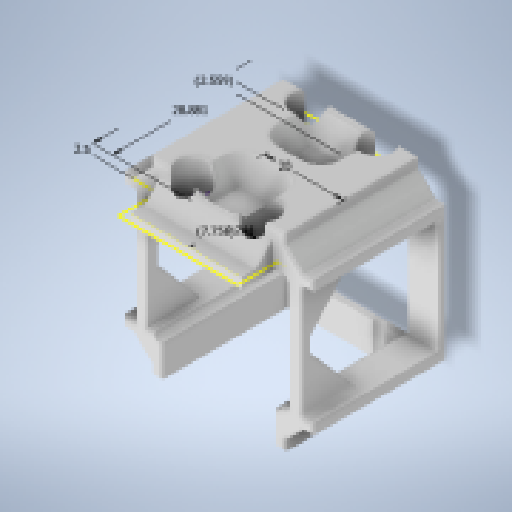
# Autodesk Inventor part: 56-spiralxy-groove-FocusToCubeAdapter
Saved by Autodesk Inventor 2024.1 (Build 281209000, 209)
## iProperties
Created: 2023-11-15
Part Number: 56-spiralxy-groove-FocusToCubeAdapter
Material: Generisch
Document SubType Name: Modeling
Designer: buchmannmartin
Density: 1 g/cm^3
Appearance: Vorgabe
Author: buchmannmartin
Autodesk Inventor part; units mm, degrees
ref_plane "YZ Plane" through (0, 0, 0) normal (1, 0, 0) x (0, 1, 0)
ref_plane "XZ Plane" through (0, 0, 0) normal (0, 1, 0) x (-1, 0, 0)
ref_plane "XY Plane" through (0, 0, 0) normal (0, 0, 1) x (1, 0, 0)
sketch "Skizze1" plane through (0, 0, 0) normal (0, 0, 1) x (1, 0, 0)
  line L0 (17.02, 23.9) -> (17.02, 21.2698) construction
  line L1 (17.02, 21.2698) -> (21.2698, 17.02) construction
  line L2 (21.2698, 17.02) -> (23.9, 17.02) construction
  line L3 (-23.9, 17.02) -> (-21.2698, 17.02) construction
  line L4 (-21.2698, 17.02) -> (-17.02, 21.2698) construction
  line L5 (-17.02, 21.2698) -> (-17.02, 23.9) construction
  line L6 (-17.02, -23.9) -> (-17.02, -21.2698) construction
  line L7 (-17.02, -21.2698) -> (-21.2698, -17.02) construction
  line L8 (-21.2698, -17.02) -> (-23.9, -17.02) construction
  line L9 (23.9, -17.02) -> (21.2698, -17.02) construction
  line L10 (21.2698, -17.02) -> (17.02, -21.2698) construction
  line L11 (17.02, -21.2698) -> (17.02, -23.9) construction
  line L12 (-14.5, 14.25) -> (14.5, 14.25)
  line L13 (16, 12.75) -> (16, -14.25)
  line L14 (14.5, -15.75) -> (-14.5, -15.75)
  line L15 (-16, -14.25) -> (-16, 12.75)
  line L16 (17.02, 23.9) -> (-17.02, 23.9) construction
  line L17 (-23.9, 17.02) -> (-23.9, -17.02) construction
  line L18 (23.9, -17.02) -> (23.9, 17.02) construction
  line L19 (17.02, -23.9) -> (-17.02, -23.9) construction
  line L20 (-16.92, 23.8) -> (-16.92, 21.2284)
  line L21 (-16.92, 21.2284) -> (-21.2284, 16.92)
  line L22 (-21.2284, 16.92) -> (-23.8, 16.92)
  line L23 (-23.8, 16.92) -> (-23.8, -16.92)
  line L24 (-23.8, -16.92) -> (-21.2284, -16.92)
  line L25 (-21.2284, -16.92) -> (-16.92, -21.2284)
  line L26 (-16.92, -21.2284) -> (-16.92, -23.8)
  line L27 (-16.92, -23.8) -> (16.92, -23.8)
  line L28 (16.92, -23.8) -> (16.92, -21.2284)
  line L29 (16.92, -21.2284) -> (21.2284, -16.92)
  line L30 (21.2284, -16.92) -> (23.8, -16.92)
  line L31 (23.8, -16.92) -> (23.8, 16.92)
  line L32 (23.8, 16.92) -> (21.2284, 16.92)
  line L33 (21.2284, 16.92) -> (16.92, 21.2284)
  line L34 (16.92, 21.2284) -> (16.92, 23.8)
  line L35 (16.92, 23.8) -> (-16.92, 23.8)
  arc A0 (16, 12.75) -> (14.5, 14.25) centre (14.5, 12.75) ccw
  arc A1 (14.5, -15.75) -> (16, -14.25) centre (14.5, -14.25) ccw
  arc A2 (-16, -14.25) -> (-14.5, -15.75) centre (-14.5, -14.25) ccw
  arc A3 (-14.5, 14.25) -> (-16, 12.75) centre (-14.5, 12.75) ccw
  point P0 (0, 0)
  point P1 (0, -15.75)
  dimension "d2" = 360
  dimension "d4" = 54.15
  dimension "d5" = 34.04
  dimension "d6" = 47.8
  dimension "d10" = 0.1
  dimension "d11" = 1.5
  dimension "d15" = 29
  dimension "d16" = 30
  dimension "d19" = 14.25
  constraints: 72 end point, 8 perpendicular, 8 point on circle, 8 tangent, 4 centre point, 4 parallel, 3 equal radius, 2 collinear, 2 horizontal, 2 vertical alignment, 1 horizontal alignment, 1 midpoint, 1 vertical, 44 other
  measures "d4" distance between parallel lines of L10 L4
  measures "d5" distance between parallel lines of L11 L6
  measures "d6" distance of L6.start L5.end
  measures "d10" distance between parallel lines of L35 L16
  measures "d11" radius of A0
  measures "d15" distance of A2.centre A1.centre
  measures "d16" distance between parallel lines of L12 L14
  measures "d19" distance from line of point (0, 0) L12
extrude "Extrusion1" add sketch "Skizze1" along normal blind 33.94
sketch "Skizze2" plane through (0, 0, 0) normal (1, 0, 0) x (0, 1, 0)
  line L0 (-15.75, 0) -> (-15.75, 33.94) construction
  line L1 (-15.75, 33.94) -> (-15.75, 38.29) construction
  line L2 (-15.75, 38.29) -> (-18.3, 38.29) construction
  line L3 (-18.3, 38.29) -> (-22.65, 33.94)
  line L4 (-22.65, 33.94) -> (-15.75, 33.94)
  line L5 (-15.75, 33.94) -> (-15.75, 41.94)
  line L6 (-15.75, 41.94) -> (-18.3, 41.94)
  line L7 (-18.3, 41.94) -> (-18.3, 38.29)
  line L8 (-0.75, 41.3732) -> (-0.75, 30.0346) construction
  line L9 (16.8, 38.29) -> (21.15, 33.94)
  line L10 (21.15, 33.94) -> (14.25, 33.94)
  line L11 (14.25, 33.94) -> (14.25, 41.94)
  line L12 (14.25, 41.94) -> (16.8, 41.94)
  line L13 (16.8, 41.94) -> (16.8, 38.29)
  line L14 (14.25, 0) -> (14.25, 33.94) construction
  line L15 (-23.8, 0) -> (-23.8, 33.94) construction
  line L16 (23.8, 0) -> (23.8, 33.94) construction
  point P0 (0, 0)
  dimension "d21" = 45
  dimension "d23" = 8
  dimension "d26" = 16.8
  dimension "d28" = 1.15
  dimension "d29" = 2.65
  constraints: 26 end point, 5 symmetric about line, 3 perpendicular, 2 vertical, 1 collinear, 1 horizontal, 1 point on line
  measures "d21" angle of L4 L3
  measures "d23" distance between parallel lines of L4 L6
  measures "d26" distance from line of L13 point (0, 0)
  measures "d28" distance from line of L3.end L15
  measures "d29" distance from line of L9.end L16
extrude "Extrusion2" add sketch "Skizze2" along normal mid plane 28 contours L9 L10 L11 L12 L13
sketch "Skizze3" plane through (-16.92, 16.8, 0) normal (0, 1, 0) x (1, 0, 0)
  line L0 (33.84, 0) -> (0, 0) construction
  line L1 (0, 0) -> (0, -33.94) construction
  line L2 (33.84, -33.94) -> (0, -33.94) construction
  line L3 (33.84, 0) -> (33.84, -33.94) construction
  line L4 (2.92, -41.94) -> (30.92, -41.94) construction
  line L5 (6.92, -14.184) -> (26.92, -14.184) construction
  line L6 (26.92, -14.184) -> (26.92, -34.184) construction
  line L7 (26.92, -34.184) -> (6.92, -34.184) construction
  line L8 (6.92, -34.184) -> (6.92, -14.184) construction
  circle A0 centre (25.67, -6.47) radius 1.7 projected
  circle A1 centre (8.17, -35.47) radius 1.7 projected
  circle A2 centre (25.67, -35.47) radius 1.7 projected
  circle A3 centre (8.17, -6.47) radius 1.7 projected
  line L9 (1.92, 2.03) -> (31.92, 2.03) projected
  line L10 (1.92, -43.97) -> (1.92, 2.03) projected
  line L11 (31.92, -43.97) -> (1.92, -43.97) projected
  line L12 (31.92, 2.03) -> (31.92, -43.97) projected
  line L13 (25.67, -31.44) -> (8.17, -31.44)
  line L14 (8.17, -31.44) -> (8.17, -2.5594)
  line L15 (8.17, -2.5594) -> (25.67, -2.5594)
  line L16 (25.67, -2.5594) -> (25.67, -31.44)
  line L17 (-4.3084, -33.94) -> (0, -33.94) projected
  point P0 (16.92, 0)
  point P1 (16.92, -14.184)
  point P2 (16.92, 0)
  point P3 (16.92, -2.5594)
  dimension "d30" = 20
  dimension "d31" = 7.756
  dimension "d32" = 0.244
  dimension "d77" = 2.5
  dimension "d78" = 28.8806
  dimension "d79" = 2.5594
  constraints: 16 end point, 4 parallel, 3 midpoint, 3 perpendicular, 2 horizontal
  measures "d30" distance of L5.start L5.end
  measures "d31" distance between parallel lines of L7 L4
  measures "d32" distance between parallel lines of L2 L7
  measures "d77" distance between parallel lines of L17 L13
  measures "d78" distance from line of point (16.92, -2.559) L13
  measures "d79" distance from line of L15 L0.end
hole "Bohrung2" at (8.75, 16.8, 2.5594) at (-8.75, 16.8, 2.5594) at (-8.75, 16.8, 31.44) at (8.75, 16.8, 31.44) direction (0, -1, 0) diameter 3.4 end through all start extended yes clearance for "Inbusschraube ISO 4762" size "M3" standard "ISO"
ref_plane "Arbeitsebene1" through (0, 0, 2.1) normal (0, 0, -1) x (-1, 0, 0)
sketch "Skizze4" plane through (0, 0, 33.94) normal (0, 0, 1) x (1, 0, 0)
  line L0 (14, 21.15) -> (14, 14.25) construction
  line L1 (14, 14.25) -> (14.5, 14.25) construction
  arc A0 (16, 12.75) -> (14.5, 14.25) centre (14.5, 12.75) ccw construction
  line L2 (16, 12.75) -> (16, -14.25) construction
  arc A1 (14.5, -15.75) -> (16, -14.25) centre (14.5, -14.25) ccw construction
  line L3 (14.5, -15.75) -> (-14.5, -15.75) construction
  arc A2 (-16, -14.25) -> (-14.5, -15.75) centre (-14.5, -14.25) ccw construction
  line L4 (-16, -14.25) -> (-16, 12.75) construction
  arc A3 (-14.5, 14.25) -> (-16, 12.75) centre (-14.5, 12.75) ccw construction
  line L5 (-14.5, 14.25) -> (-14, 14.25) construction
  line L6 (-14, 14.25) -> (-14, 21.15) construction
  line L7 (-14, 21.15) -> (14, 21.15) construction
  line L8 (-16.92, 21.2284) -> (-21.2284, 16.92) construction
  line L9 (-21.2284, 16.92) -> (-23.8, 16.92) construction
  line L10 (-23.8, 16.92) -> (-23.8, -16.92) construction
  line L11 (-23.8, -16.92) -> (-21.2284, -16.92) construction
  line L12 (-21.2284, -16.92) -> (-16.92, -21.2284) construction
  line L13 (-16.92, -21.2284) -> (-16.92, -23.8) construction
  line L14 (-16.92, -23.8) -> (16.92, -23.8) construction
  line L15 (16.92, -23.8) -> (16.92, -21.2284) construction
  line L16 (16.92, -21.2284) -> (21.2284, -16.92) construction
  line L17 (21.2284, -16.92) -> (23.8, -16.92) construction
  line L18 (23.8, -16.92) -> (23.8, 16.92) construction
  line L19 (23.8, 16.92) -> (21.2284, 16.92) construction
  line L20 (21.2284, 16.92) -> (16.92, 21.2284) construction
  line L21 (16.92, 21.2284) -> (16.92, 23.8) construction
  line L22 (16.92, 23.8) -> (-16.92, 23.8) construction
  line L23 (-16.92, 23.8) -> (-16.92, 21.2284) construction
  line L24 (-23.8, -14.25) -> (23.8, -14.25)
  line L25 (23.8, -14.25) -> (23.8, 14.25)
  line L26 (23.8, 14.25) -> (-23.8, 14.25)
  line L27 (-23.8, 14.25) -> (-23.8, -14.25)
  line L28 (-14.25, -23.8) -> (14.25, -23.8)
  line L29 (14.25, -23.8) -> (14.25, -14.25)
  line L30 (14.25, -14.25) -> (-14.25, -14.25)
  line L31 (-14.25, -14.25) -> (-14.25, -23.8)
  point P0 (0, 0)
  point P1 (0, -14.25)
  point P2 (0, -14.25)
  point P3 (-23.8, 0)
  point P4 (-14.25, 14.25)
  constraints: 16 end point, 5 midpoint, 4 parallel, 3 perpendicular, 2 horizontal, 2 point on line, 1 coincident, 1 collinear, 1 vertical alignment
extrude "Extrusion3" cut sketch "Skizze4" against normal up to surface (31.84 mm away)
sketch "Skizze5" plane through (0, 0, 0) normal (1, 0, 0) x (0, 1, 0)
  line L0 (-14.25, 2.1) -> (-14.25, 33.94) construction
  line L1 (14.25, 33.94) -> (14.25, 2.1) construction
  line L2 (-14.25, 33.94) -> (14.25, 33.94)
  line L3 (14.25, 33.94) -> (14.25, 20.1)
  line L4 (14.25, 20.1) -> (2, 30.94)
  line L5 (2, 30.94) -> (-2, 30.94)
  line L6 (-2, 30.94) -> (-14.25, 20.1)
  line L7 (-14.25, 20.1) -> (-14.25, 33.94)
  point P0 (0, 0)
  point P1 (0, 30.94)
  point P2 (0, 33.94)
  dimension "d53" = 4
  dimension "d54" = 3
  dimension "d55" = 18
  dimension "d56" = 48.495
  constraints: 12 end point, 2 collinear, 2 midpoint, 1 horizontal, 1 horizontal alignment, 1 parallel, 1 perpendicular, 1 vertical alignment
  measures "d53" distance of L4.end L5.end
  measures "d54" distance between parallel lines of L2 L5
  measures "d55" distance of L1.end L3.end
  measures "d56" angle of L1 L4
extrude "Extrusion4" add sketch "Skizze5" against normal blind 6 from surface at 23.8
extrude "Extrusion5" cut sketch "Skizze5" against normal blind 3 from surface at 23.8
pattern_circular "Runde Anordnung1" count 2 over 360 about axis through (0, 0, -10) along (0, 0, -1) of "Extrusion4", "Extrusion5"
fillet "Rundung1" radius 1 4 edges at (20.8, -14.25, 27.02) (17.8, -14.25, 27.02) (20.8, 14.25, 27.02) (17.8, 14.25, 27.02)
sketch "Skizze6" plane through (-16.92, 23.8, 0) normal (0, 1, 0) x (1, 0, 0)
  arc A0 (25.4144, -37.1507) -> (27.1756, -36.2593) centre (26.92, -37.94) ccw construction
  circle A1 centre (6.92, -17.94) radius 1.7 construction
  line L0 (19.8489, -35.8689) -> (13.9911, -35.8689)
  line L1 (8.9911, -30.8689) -> (8.9911, -25.0111)
  line L2 (13.9911, -20.0111) -> (19.8489, -20.0111)
  line L3 (24.8489, -25.0111) -> (24.8489, -30.8689)
  arc A2 (19.8489, -35.8689) -> (24.8489, -30.8689) centre (19.8489, -30.8689) ccw
  arc A3 (24.8489, -25.0111) -> (19.8489, -20.0111) centre (19.8489, -25.0111) ccw
  arc A4 (13.9911, -20.0111) -> (8.9911, -25.0111) centre (13.9911, -25.0111) ccw
  line L4 (32.92, -2.1) -> (40.72, -2.1) construction
  arc A5 (8.9911, -30.8689) -> (13.9911, -35.8689) centre (13.9911, -30.8689) ccw
  line L5 (13.9911, -30.8689) -> (19.8489, -25.0111) construction
  line L6 (19.8489, -30.8689) -> (13.9911, -25.0111) construction
  circle A6 centre (6.92, -17.94) radius 4 construction
  line L7 (26.92, -37.94) -> (6.92, -17.94) construction
  line L8 (6.92, -17.94) -> (26.92, -17.94) construction
  line L9 (16.92, 0) -> (16.92, -17.94) construction
  line L10 (19.8489, -15.8689) -> (13.9911, -15.8689)
  line L11 (8.9911, -10.8689) -> (8.9911, -7.1)
  line L12 (13.9911, -2.1) -> (19.8489, -2.1)
  line L13 (24.8489, -7.1) -> (24.8489, -10.8689)
  arc A7 (19.8489, -15.8689) -> (24.8489, -10.8689) centre (19.8489, -10.8689) ccw
  arc A8 (24.8489, -7.1) -> (19.8489, -2.1) centre (19.8489, -7.1) ccw
  arc A9 (13.9911, -2.1) -> (8.9911, -7.1) centre (13.9911, -7.1) ccw
  arc A10 (8.9911, -10.8689) -> (13.9911, -15.8689) centre (13.9911, -10.8689) ccw
  line L14 (19.8489, -10.8689) -> (13.9911, -7.1) construction
  point P0 (16.92, -27.94)
  point P1 (16.92, -8.9845)
  dimension "d65" = 5
  dimension "d67" = 1
  constraints: 28 end point, 16 point on circle, 16 tangent, 8 centre point, 7 equal radius, 6 midpoint, 4 parallel, 3 horizontal, 3 perpendicular, 2 collinear, 1 point on line, 1 vertical alignment, 1 other
  measures "d65" radius of A2
extrude "Extrusion6" cut sketch "Skizze6" against normal blind 5 draft -40
chamfer "Fasen1" distance 2 angle 45 5 edges at (0, 21.5012, 33.94) (-4.65, 22.0367, 33.94) (4.65, 22.0367, 33.94) (14, 15.525, 41.94) (-14, 15.525, 41.94)
chamfer "Fasen2" distance 0.5 angle 45 72 edges at (23.8, 0, 0) (22.5142, -16.92, 0) (19.0742, -19.0742, 0) (16.92, -22.5142, 0) (0, -23.8, 0) (-16.92, -22.5142, 0) (-19.0742, -19.0742, 0) (-22.5142, -16.92, 0) (-23.8, 0, 0) (-22.5142, 16.92, 0) (-19.0742, 19.0742, 0) (-16.92, 22.5142, 0) (0, 23.8, 0) (16.92, 22.5142, 0) (19.0742, 19.0742, 0) (22.5142, 16.92, 0) (22.8, 14.25, 33.94) (21.0929, 13.9571, 33.94) (20.8, 0, 33.94) (21.0929, -13.9571, 33.94) (22.8, -14.25, 33.94) (23.8, 15.585, 33.94) (22.5142, 16.92, 33.94) (19.0742, 19.0742, 33.94) (16.92, 22.5142, 33.94) (13.3155, 23.8, 33.94) (-13.3155, 23.8, 33.94) (-16.92, 22.5142, 33.94) (-19.0742, 19.0742, 33.94) (-22.5142, 16.92, 33.94) (-23.8, 15.585, 33.94) (-22.3, 14.25, 33.94) (-15.9, 14.25, 33.94) (15.4, 14.25, 33.94) (-22.3, -14.25, 33.94) (-16.9, -14.25, 33.94) (16.4, -14.25, 33.94) (-23.8, -15.585, 33.94) (-22.5142, -16.92, 33.94) (-19.0742, -19.0742, 33.94) (-16.92, -22.5142, 33.94) (-15.585, -23.8, 33.94) (-14.25, -19.775, 33.94) (-20.8, 0, 33.94) (14.25, -19.775, 33.94) (16.92, -22.5142, 33.94) (15.585, -23.8, 33.94) (19.0742, -19.0742, 33.94) (23.8, -15.585, 33.94) (22.5142, -16.92, 33.94) (0, 14.25, 0) (15.5607, 13.8107, 0) (16, -0.75, 0) (15.5607, -15.3107, 0) (0, -15.75, 0) (-15.5607, -15.3107, 0) (-16, -0.75, 0) (-15.5607, 13.8107, 0) (-20.8, 8.125, 25.52) (-17.8, 8.125, 25.52) (-20.8, -8.125, 25.52) (-17.8, -8.125, 25.52) (20.8, 7.625, 25.9624) (21.0929, 13.9571, 20.3592) (17.8, 7.625, 25.9624) (17.5071, 13.9571, 20.3592) (20.8, 0, 30.94) (17.8, -7.625, 25.9624) (17.5071, -13.9571, 20.3592) (20.8, -7.625, 25.9624) (21.0929, -13.9571, 20.3592) (17.8, 0, 30.94)
sketch "Skizze7" plane through (-2.9289, 23.8, 20.0111) normal (0, 1, 0) x (1, 0, 0)
  line L0 (0, 17.9111) -> (5.8579, 17.9111) projected
  arc A0 (10.8579, 12.9111) -> (5.8579, 17.9111) centre (5.8579, 12.9111) ccw projected
  line L1 (10.8579, 12.9111) -> (10.8579, 9.1421) projected
  arc A1 (5.8579, 4.1421) -> (10.8579, 9.1421) centre (5.8579, 9.1421) ccw projected
  line L2 (5.8579, 4.1421) -> (0, 4.1421) projected
  arc A2 (-5, 9.1421) -> (0, 4.1421) centre (0, 9.1421) ccw projected
  line L3 (-5, 9.1421) -> (-5, 12.9111) projected
  arc A3 (0, 17.9111) -> (-5, 12.9111) centre (0, 12.9111) ccw projected
  circle A4 centre (-5.8211, 17.4517) radius 1.7 projected
  circle A5 centre (11.6789, 17.4517) radius 1.7 projected
  line L4 (-6.3058, -13.4289) -> (-13.9911, -13.4289) projected
  arc A6 (-5, -9.9404) -> (-5.9745, -13.122) centre (-5.8211, -11.4289) ccw projected
  line L5 (-5, -9.9404) -> (-5, -5) projected
  arc A7 (0, 0) -> (-5, -5) centre (0, -5) ccw projected
  line L6 (0, 0) -> (5.8579, 0) projected
  arc A8 (10.8579, -5) -> (5.8579, 0) centre (5.8579, -5) ccw projected
  line L7 (10.8579, -5) -> (10.8579, -9.9404) projected
  arc A9 (11.8324, -13.122) -> (10.8579, -9.9404) centre (11.6789, -11.4289) ccw projected
  line L8 (19.8489, -13.4289) -> (12.1637, -13.4289) projected
  line L9 (19.8489, 19.5111) -> (19.8489, -13.4289) projected
  line L10 (-13.9911, 19.5111) -> (19.8489, 19.5111) projected
  line L11 (-13.9911, 19.5111) -> (-13.9911, -13.4289) projected
  line L12 (12.0918, -12.1441) -> (11.2661, -12.1441)
  line L13 (11.2661, -12.1441) -> (10.8532, -11.4289)
  line L14 (10.8532, -11.4289) -> (11.2661, -10.7138)
  line L15 (11.2661, -10.7138) -> (12.0918, -10.7138)
  line L16 (12.0918, -10.7138) -> (12.5047, -11.4289)
  line L17 (12.5047, -11.4289) -> (12.0918, -12.1441)
  circle A10 centre (-5.8211, -11.4289) radius 1.7 projected
  line L18 (-4.0024, -8.2789) -> (-2.1838, -11.4289)
  line L19 (-2.1838, -11.4289) -> (-4.0024, -14.5789)
  line L20 (-4.0024, -14.5789) -> (-7.6397, -14.5789)
  line L21 (-7.6397, -14.5789) -> (-9.4584, -11.4289)
  line L22 (-9.4584, -11.4289) -> (-7.6397, -8.2789)
  line L23 (-7.6397, -8.2789) -> (-4.0024, -8.2789)
  line L24 (9.8603, 20.6017) -> (13.4976, 20.6017)
  line L25 (13.4976, 20.6017) -> (15.3162, 17.4517)
  line L26 (15.3162, 17.4517) -> (13.4976, 14.3017)
  line L27 (13.4976, 14.3017) -> (9.8603, 14.3017)
  line L28 (9.8603, 14.3017) -> (8.0416, 17.4517)
  line L29 (8.0416, 17.4517) -> (9.8603, 20.6017)
  line L30 (19.8489, -13.4289) -> (12.1637, -13.4289) projected
  line L31 (-6.3058, -13.4289) -> (-13.9911, -13.4289) projected
  line L32 (9.8603, -8.2789) -> (13.4976, -8.2789)
  line L33 (13.4976, -8.2789) -> (15.3162, -11.4289)
  line L34 (15.3162, -11.4289) -> (13.4976, -14.5789)
  line L35 (13.4976, -14.5789) -> (9.8603, -14.5789)
  line L36 (9.8603, -14.5789) -> (8.0416, -11.4289)
  line L37 (8.0416, -11.4289) -> (9.8603, -8.2789)
  line L38 (-7.6397, 20.6017) -> (-4.0024, 20.6017)
  line L39 (-4.0024, 20.6017) -> (-2.1838, 17.4517)
  line L40 (-2.1838, 17.4517) -> (-4.0024, 14.3017)
  line L41 (-4.0024, 14.3017) -> (-7.6397, 14.3017)
  line L42 (-7.6397, 14.3017) -> (-9.4584, 17.4517)
  line L43 (-9.4584, 17.4517) -> (-7.6397, 20.6017)
  point P0 (11.6789, 20.6017)
  point P1 (11.6789, 14.3017)
  dimension "d80" = 6.3
  dimension "d81" = 6.3
  constraints: 60 end point, 5 coincident, 2 midpoint, 2 parallel, 1 collinear, 67 other
  measures "d80" distance between parallel lines of L23 L20
  measures "d81" distance of point (11.679, 20.602) point (11.679, 14.302)
extrude "Extrusion7" cut sketch "Skizze7" against normal blind 5 contours L40 L41 A3 | A3 L41 L42 L43 L10 L39 L40 | L28 L29 L10 L25 L26 L27 A0 | A0 L27 L28 | L10 L43 L38 L39 | L29 L24 L25 L10 | L21 L22 L23 L18 L19 L20 | L34 L35 L36 L37 L32 L33 | A4 | A5 | A10 A6 | L12 L13 L14 L15 L16 L17
